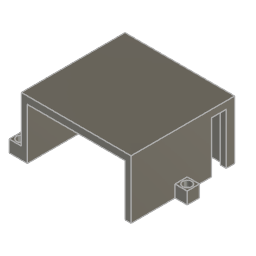
Cache Moteur 2 (Autodesk Fusion 360 design; units mm, degrees)
Autodesk Fusion 360 part; units mm, degrees
note: some values were not read from the file. Set by a fixed rule: which sketch regions a step uses.
sketch "Esquisse1" plane through (0, 0, 0) normal (0, 0, 1) x (1, 0, 0)
  line L0 (-22.5, 21.25) -> (22.5, 21.25)
  line L1 (22.5, 21.25) -> (22.5, -21.25)
  line L2 (22.5, -21.25) -> (-22.5, -21.25)
  line L3 (-22.5, -21.25) -> (-22.5, 21.25)
  line L4 (-22.5, 21.25) -> (22.5, -21.25) construction
  line L5 (22.5, 21.25) -> (-22.5, -21.25) construction
  line L6 (-22.5, 11.75) -> (-22.5, 21.25)
  line L7 (-22.5, -21.25) -> (-27.5, -21.25)
  line L8 (-27.5, -21.25) -> (-27.5, -16.25)
  line L9 (-27.5, -16.25) -> (-22.5, -16.25)
  line L10 (-22.5, -16.25) -> (-22.5, -21.25)
  line L11 (22.5, 21.25) -> (27.5, 21.25)
  line L12 (27.5, 21.25) -> (27.5, 16.25)
  line L13 (27.5, 16.25) -> (22.5, 16.25)
  line L14 (22.5, 16.25) -> (22.5, 21.25)
  line L15 (22.5, -21.25) -> (27.5, -21.25)
  line L16 (27.5, -21.25) -> (27.5, -16.25)
  line L17 (27.5, -16.25) -> (22.5, -16.25)
  line L18 (22.5, -16.25) -> (22.5, -21.25)
  line L19 (-20, -21.25) -> (20, -21.25)
  line L20 (20, -21.25) -> (20, 18.75)
  line L21 (20, 18.75) -> (-20, 18.75)
  line L22 (-20, 18.75) -> (-20, -21.25)
  line L23 (22.5, 21.25) -> (27.5, 16.25)
  line L24 (22.5, -16.25) -> (27.5, -21.25)
  line L25 (-27.5, -16.25) -> (-22.5, -21.25)
  circle A0 centre (25, 18.75) radius 1.9
  circle A1 centre (25, 18.75) radius 1
  circle A2 centre (25, -18.75) radius 1.9
  circle A3 centre (25, -18.75) radius 1
  circle A4 centre (-25, -18.75) radius 1.9
  circle A5 centre (-25, -18.75) radius 1
  line L26 (27.5, 21.25) -> (27.5, 16.25)
  circle A6 centre (25, 18.75) radius 1
  line L27 (-22.5, 21.25) -> (-27.5, 21.25)
  line L28 (-27.5, 21.25) -> (-27.5, 16.25)
  line L29 (-27.5, 16.25) -> (-22.5, 16.25)
  line L30 (-22.5, 16.25) -> (-22.5, 21.25)
  circle A7 centre (-25, 18.75) radius 1.9
  circle A8 centre (-25, 18.75) radius 1
  line L31 (-22.5, 16.25) -> (-27.5, 21.25)
  line L32 (27.5, 1.75) -> (22.5, 1.75)
  line L33 (22.5, 1.75) -> (27.5, -3.25)
  circle A9 centre (25, -0.75) radius 1
  circle A10 centre (25, -0.75) radius 1.9
  line L34 (27.5, -3.25) -> (27.5, 1.75)
  line L35 (22.5, -3.25) -> (27.5, -3.25)
  point P0 (25, 18.75)
  point P1 (-25, 18.75)
  dimension "d1" = 45
  dimension "d2" = 42.5
  dimension "d5" = 5
  dimension "d6" = 5
  dimension "d7" = 5
  dimension "d8" = 5
  dimension "d9" = 5
  dimension "d10" = 5
  dimension "d12" = 2.5
  dimension "d13" = 2.5
  dimension "d14" = 2.5
  dimension "d22" = 3.8
  dimension "d23" = 2
  dimension "d26" = 3.8
  dimension "d27" = 2
  dimension "d28" = 3.8
  dimension "d29" = 2
  dimension "d46" = 5
  dimension "d47" = 2
  dimension "d48" = 5
  dimension "d49" = 5
  dimension "d50" = 2
  dimension "d51" = 3.8
  dimension "d52" = 5
  dimension "d53" = 5
  dimension "d54" = 3.8
  dimension "d55" = 2
  dimension "d56" = 13
  constraint horizontal L0
  constraint perpendicular L0 L1
  constraint parallel L0 L2
  constraint parallel L1 L3
  constraint coincident L4 origin
  constraint coincident L5 origin
  constraint vertical L6
  constraint horizontal L7
  constraint vertical L8
  constraint horizontal L9
  constraint vertical L10
  constraint horizontal L11
  constraint vertical L12
  constraint horizontal L13
  constraint vertical L14
  constraint horizontal L15
  constraint vertical L16
  constraint horizontal L17
  constraint vertical L18
  constraint horizontal L19
  constraint vertical L20
  constraint horizontal L21
  constraint vertical L22
  constraint coincident L2 L19.start
  constraint midpoint L23 P0
  constraint concentric A0 A1
  constraint midpoint L24 A2.centre
  constraint concentric A2 A3
  constraint midpoint L25 A4.centre
  constraint concentric A4 A5
  constraint vertical L26
  constraint horizontal L27
  constraint vertical L28
  constraint horizontal L29
  constraint vertical L30
  constraint concentric A7 A8
  constraint midpoint L31 P1
  constraint coincident P1 A7.centre
  constraint horizontal L35
  constraint vertical L34
  constraint horizontal L32
  constraint midpoint A9.centre L33
  constraint concentric A9 A10
  constraint coincident L1 L32.end
  constraint coincident L1 L35.start
  measures "d1" distance of L0.start L0.end
  measures "d2" distance of L0.start L2.end
  measures "d5" distance of L7.end L8.end
  measures "d6" distance of L8.end L9.end
  measures "d7" distance of L11.end L12.end
  measures "d8" distance of L12.end L13.end
  measures "d9" distance of L15.end L16.end
  measures "d10" distance of L1.end L15.end
  measures "d12" distance of L0 L21
  measures "d13" distance of L3 L22
  measures "d14" distance of L1 L20
  measures "d22" diameter of A4
  measures "d23" diameter of A5
  measures "d26" diameter of A0
  measures "d27" diameter of A1
  measures "d28" diameter of A2
  measures "d29" diameter of A3
  measures "d46" distance of L12.end L11.end
  measures "d47" diameter of A6
  measures "d48" distance of L28.end L29.end
  measures "d49" distance of L27.end L28.end
  measures "d50" diameter of A8
  measures "d51" diameter of A7
  measures "d52" distance of L32.start L33.end
  measures "d53" distance of L35.start L33.end
  measures "d54" diameter of A10
  measures "d55" diameter of A9
  measures "d56" distance of L17 L35
extrude "Extrusion1" add sketch "Esquisse1" along normal blind 24 contours L0 L1 L2 L3 L6 L10 L14 L18 L20 L21 L22 L30
extrude "Extrusion2" add sketch "Esquisse1" along normal blind 3 from surface at 21 contours L2 L19 L20 L21 L22
extrude "Extrusion3" add sketch "Esquisse1" along normal blind 5 contours L3 L6 L27 L30 A7 L31 | L28 L29 A7 L31 | A7 A8 L31 | A7 A8 L31 | L1 L33 A10 L35 | L32 L33 A10 L34 | L3 L9 L10 L25 A4 | A8 L31 | A8 L31 | L33 A9 A10 | L33 A9 A10 | L7 L8 L25 A4 | L33 A9 | L33 A9 | L25 A4 A5 | L25 A4 A5 | L25 A5 | L25 A5
extrude "Extrusion4" cut sketch "Esquisse1" against normal blind 2.5 from surface at 5 contours L23 A0 A1 A6 | L23 A0 A1 A6 | A7 A8 L31 | A7 A8 L31 | L33 A9 A10 | L33 A9 A10 | L25 A4 A5 | L25 A4 A5 | L24 A2 A3 | L24 A2 A3
extrude "Extrusion5" cut sketch "Esquisse1" along normal blind 8 contours A8 L31 | A8 L31 | L33 A9 | L33 A9 | L25 A5 | L25 A5 | L24 A3 | L24 A3
sketch "Esquisse2" plane through (-22.5, 0, 0) normal (-1, 0, 0) x (0, -1, 0)
  line L0 (16.25, 5) -> (21.25, 5)
  line L1 (21.25, 5) -> (21.25, 24)
  line L2 (21.25, 24) -> (-21.25, 24)
  line L3 (-21.25, 24) -> (-21.25, 5)
  line L4 (-16.25, 0) -> (16.25, 0)
  line L5 (16.25, 0) -> (16.25, 5)
  line L6 (-17.75, 0) -> (-17.75, 21)
  line L7 (-11.75, 0) -> (-11.75, 21)
  line L8 (-17.75, 21) -> (-11.75, 21)
  line L9 (-21.25, 5) -> (-16.25, 5)
  line L10 (-16.25, 5) -> (-16.25, 0)
  line L11 (-11.75, 0) -> (-17.75, 0)
  dimension "d35" = 3.5
  dimension "d36" = 6
  dimension "d37" = 21
  dimension "d38" = 21
  constraint coincident L4 L6.start
  constraint perpendicular L4 L6
  constraint coincident L4 L7.start
  constraint perpendicular L4 L7
  measures "d35" distance of L3 L6
  measures "d36" distance of L6 L7
  measures "d37" distance of L6.start L6.end
  measures "d38" distance of L7.start L7.end
extrude "Extrusion6" cut sketch "Esquisse2" against normal blind 9 from surface at -40 contours L4 L6 L7 L8 L9 L10 L11 | L6 L9 L10 L11
sketch "Esquisse3" plane through (22.5, 0, 0) normal (1, 0, 0) x (0, 1, 0)
  line L0 (17.75, 0) -> (21.25, 0)
  line L1 (21.25, 0) -> (21.25, 24)
  line L2 (17.75, 0) -> (27.75, 0)
  line L3 (27.75, 0) -> (27.75, 21)
  line L4 (27.75, 21) -> (17.75, 21)
  line L5 (17.75, 21) -> (17.75, 0)
  line L6 (17.75, 21) -> (17.75, 0)
  line L7 (11.75, 0) -> (11.75, 21)
  line L8 (11.75, 21) -> (17.75, 21)
  line L9 (21.25, 24) -> (-21.25, 24)
  line L10 (-21.25, 24) -> (-21.25, 0)
  line L11 (-3.25, 5) -> (1.75, 5)
  line L12 (1.75, 0) -> (11.75, 0)
  line L13 (-21.25, 0) -> (-3.25, 0)
  line L14 (-3.25, 0) -> (-3.25, 5)
  line L15 (1.75, 5) -> (1.75, 0)
  dimension "d41" = 10
  dimension "d42" = 21
  constraint horizontal L2
  constraint vertical L3
  constraint horizontal L4
  constraint vertical L5
  constraint coincident L0.start L2.start
  measures "d41" distance of L3.end L4.end
  measures "d42" distance of L2.end L3.end
